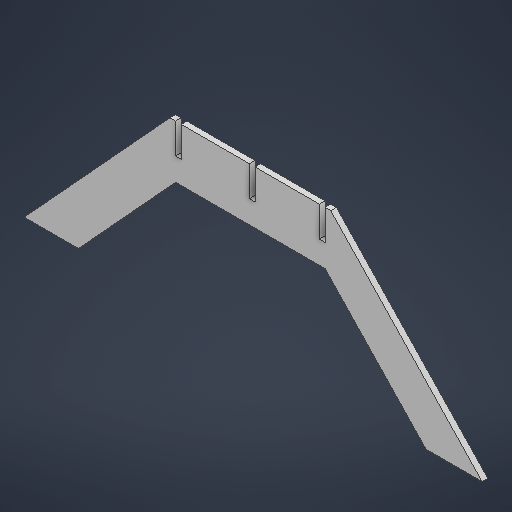
# Autodesk Inventor part: Base
Saved by Autodesk Inventor 2027 (Build 310192000, 192)
## iProperties
Created: 2026-05-24
Part Number: Base
Material: Generic
Document SubType Name: Modeling
Designer: alexy
Density: 1 g/cm^3
Appearance: Default
Author: alexy
Autodesk Inventor part; units mm, degrees
ref_plane "YZ Plane" through (0, 0, 0) normal (1, 0, 0) x (0, 1, 0)
ref_plane "XZ Plane" through (0, 0, 0) normal (0, 1, 0) x (-1, 0, 0)
ref_plane "XY Plane" through (0, 0, 0) normal (0, 0, 1) x (1, 0, 0)
sketch "Sketch1" plane through (0, 0, 0) normal (0, 0, 1) x (1, 0, 0)
  line L0 (0, 0) -> (0, 16)
  line L1 (0, 16) -> (0, 16)
  line L2 (0, 16) -> (0, 0)
  line L3 (0, 0) -> (3, 0)
  line L4 (3, 0) -> (3, 16)
  line L5 (3, 16) -> (6, 16)
  line L6 (6, 16) -> (86, -68)
  line L7 (86, -68) -> (-156, -68)
  line L8 (-73, 16) -> (-73, 0)
  line L9 (-73, 0) -> (-76, 0)
  line L10 (-76, 0) -> (-76, 16)
  line L11 (-127.3333, -68) -> (-76, -12)
  line L12 (-76, -12) -> (3, -12)
  line L13 (3, -12) -> (56.3333, -68)
  line L14 (-76, 16) -> (-79, 16)
  line L15 (-79, 16) -> (-156, -68)
  line L16 (-73, 16) -> (-37, 16)
  line L17 (-37, 16) -> (-37, 0)
  line L18 (-37, 0) -> (-34, 0)
  line L19 (-34, 0) -> (-34, 16)
  line L20 (-34, 16) -> (0, 16)
  point P0 (1.5, 0)
  dimension "d0" = 3
  dimension "d1" = 16
  dimension "d2" = 3
  dimension "d8" = 3
  dimension "d9" = 80
  dimension "d10" = 80
  dimension "d12" = 12
  dimension "d13" = 3
  dimension "d14" = 56
  dimension "d15" = 3
  dimension "d16" = 34
  dimension "d17" = 36
  constraints: 42 end point, 9 perpendicular, 4 horizontal alignment, 4 point on line, 3 horizontal, 3 parallel, 3 vertical, 3 vertical alignment, 1 coincident, 1 midpoint
  measures "d0" distance of L2.end L3.end
  measures "d1" distance of L3.end L4.end
  measures "d2" distance of L4.end L5.end
  measures "d8" distance of L8.end L9.end
  measures "d9" horizontal distance of L7.end L10.end
  measures "d10" horizontal distance of L6.end L5.end
  measures "d12" distance between parallel lines of L12 L9
  measures "d13" distance of L10.end L14.end
  measures "d14" distance between parallel lines of L7 L12
  measures "d15" distance of L17.end L18.end
  measures "d16" distance of L19.end L1.end
  measures "d17" distance of L8.start L16.end
extrude "Extrusion1" add sketch "Sketch1" along normal blind 3 contours L3 L4 L5 L6 L7 L13 L12 L11 L15 L14 L10 L9 L8 L16 L17 L18 L19 L20 L0
body "Solid1"
